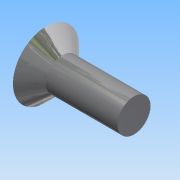
# Autodesk Inventor part: fraisee
Saved by Autodesk Inventor 2015 (Build 190159000, 159)
## iProperties
Created: 2016-04-17
Part Number: fraisee
Material: Générique
Document SubType Name: Modeling
Designer: Gregwar
Density: 1 g/cm^3
Appearance: Par défaut
Author: Gregwar
Autodesk Inventor part; units mm, degrees
ref_plane "YZ Plane" through (0, 0, 0) normal (1, 0, 0) x (0, 1, 0)
ref_plane "XZ Plane" through (0, 0, 0) normal (0, 1, 0) x (-1, 0, 0)
ref_plane "XY Plane" through (0, 0, 0) normal (0, 0, 1) x (1, 0, 0)
sketch "Esquisse1" plane through (0, 0, 0) normal (0, 1, 0) x (-1, 0, 0)
  line L0 (0, 0) -> (8, 0)
  line L1 (8, 0) -> (8, -3)
  line L2 (8, -3) -> (6.5, -1.5)
  line L3 (6.5, -1.5) -> (0, -1.5)
  line L4 (0, -1.5) -> (0, 0)
  line L5 (8, 0) -> (8, 3)
  line L6 (8, 3) -> (6.5, 1.5)
  line L7 (6.5, 1.5) -> (0, 1.5)
  line L8 (0, 1.5) -> (0, 0)
  dimension "d0" = 90
  dimension "d1" = 3
  dimension "d2" = 6
  dimension "d3" = 8
  constraints: 18 end point, 3 symmetric about line, 2 perpendicular, 1 horizontal, 1 parallel
  measures "d0" angle of L6 L2
  measures "d1" distance of L7.end L3.end
  measures "d2" distance of L1.end L5.end
  measures "d3" distance between parallel lines of L4 L1
revolve "Révolution1" add sketch "Esquisse1" angle 360 about axis through (0, 0, 0) along (-1, 0, 0) contours L0 L1 L2 L3 L4
sketch "Esquisse2" plane through (-8, 0, 0) normal (-1, 0, 0) x (0, 0, 1)
  line L0 (0.7217, 1.25) -> (1.4434, 0)
  line L1 (1.4434, 0) -> (0.7217, -1.25)
  line L2 (0.7217, -1.25) -> (-0.7217, -1.25)
  line L3 (-0.7217, -1.25) -> (-1.4434, 0)
  line L4 (-1.4434, 0) -> (-0.7217, 1.25)
  line L5 (-0.7217, 1.25) -> (0.7217, 1.25)
  point P0 (0, 0)
  point P1 (0, 0)
  dimension "d5" = 2.5
  constraints: 12 end point, 1 coincident, 1 horizontal, 13 other
  measures "d5" distance between parallel lines of L2 L5
extrude "Extrusion1" cut sketch "Esquisse2" against normal blind 1
